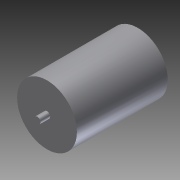
# Autodesk Inventor part: RS775 18v
Saved by Autodesk Inventor 2011 SP1 (Build 150282100, 282)
## iProperties
Created: 2013-01-16
Part Number: RS775 18v
Document SubType Name: Modeling
Designer: 961407
Density: 1 g/cm^3
Author: 961407
Autodesk Inventor part; units mm, degrees
ref_plane "YZ Plane" through (0, 0, 0) normal (1, 0, 0) x (0, 1, 0)
ref_plane "XZ Plane" through (0, 0, 0) normal (0, 1, 0) x (-1, 0, 0)
ref_plane "XY Plane" through (0, 0, 0) normal (0, 0, 1) x (1, 0, 0)
sketch "Sketch1" plane through (0, 0, 0) normal (0, 0, 1) x (1, 0, 0)
  circle A0 centre (0, 0) radius 23.495
  dimension "d0" = 46.99
  constraints: 1 centre point, 1 coincident
  measures "d0" diameter of A0
extrude "Extrusion1" add sketch "Sketch1" against normal blind 71.374
sketch "Sketch2" plane through (0, 0, 0) normal (0, 0, 1) x (1, 0, 0)
  circle A0 centre (0, 0) radius 23.495 projected
  circle A1 centre (0, 0) radius 2.54
  dimension "d3" = 5.08
  constraints: 1 centre point, 1 coincident
  measures "d3" diameter of A1
extrude "Extrusion2" add sketch "Sketch2" along normal blind 7.62 contours A1
sketch "Sketch3" plane through (0, 0, -71.374) normal (0, 0, -1) x (-1, 0, 0)
  circle A0 centre (0, 0) radius 23.495 projected
  line L0 (-13.081, 1.651) -> (-12.7, 1.651)
  line L1 (-12.7, 1.651) -> (-12.7, -1.651)
  line L2 (-12.7, -1.651) -> (-13.081, -1.651)
  line L3 (-13.081, -1.651) -> (-13.081, 1.651)
  line L4 (12.7, 1.651) -> (13.081, 1.651)
  line L5 (13.081, 1.651) -> (13.081, -1.651)
  line L6 (13.081, -1.651) -> (12.7, -1.651)
  line L7 (12.7, -1.651) -> (12.7, 1.651)
  dimension "d6" = 3.302
  dimension "d7" = 3.302
  dimension "d8" = 0.381
  dimension "d9" = 0.381
  dimension "d10" = 1.651
  dimension "d11" = 0
  dimension "d12" = 25.4
  dimension "d13" = 12.7
  constraints: 16 end point, 4 parallel, 2 horizontal, 2 perpendicular
  measures "d6" distance of L0.end L1.end
  measures "d7" distance of L4.end L5.end
  measures "d8" distance of L1.end L2.end
  measures "d9" distance of L5.end L6.end
  measures "d10" distance from line of L4 A0.centre
  measures "d11" distance between parallel lines of L4 L0
  measures "d12" distance between parallel lines of L7 L1
  measures "d13" distance from line of L7 A0.centre
extrude "Extrusion3" add sketch "Sketch3" along normal blind 3.81 contours L0 L1 L2 L3 | L4 L5 L6 L7
sketch "Sketch4" plane through (-13.081, -1.651, -71.374) normal (-1, 0, 0) x (0, 0, 1)
  line L0 (0, 3.302) -> (-3.81, 3.302) projected
  circle A0 centre (-1.905, 1.651) radius 0.9525
  point P0 (71.374, 1.651)
  dimension "d16" = 1.905
  dimension "d17" = 0.6985
  constraints: 1 centre point
  measures "d16" diameter of A0
  measures "d17" distance edge to line of A0 L0
extrude "Extrusion4" cut sketch "Sketch4" against normal blind 127
body "Solid1"
